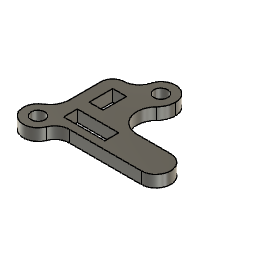
part_A25 (Autodesk Fusion 360 design; units mm, degrees)
Autodesk Fusion 360 part; units mm, degrees
sketch "Sketch1" plane through (0, 0, 0) normal (0, 0, 1) x (1, 0, 0)
  line L0 (0, 0) -> (35, 0)
  line L1 (35, 0) -> (35, 40)
  line L2 (35, 40) -> (0, 40)
  line L3 (0, 40) -> (0, 0)
  dimension "d1" = 35
  dimension "d2" = 40
  constraint horizontal L0
  constraint vertical L1
  constraint horizontal L2
  constraint vertical L3
  constraint coincident L0.start L3.end
  measures "d1" distance of L0.start L0.end
  measures "d2" distance of L0.start L2.end
extrude "Extrude1" add sketch "Sketch1" along normal blind 3
sketch "Sketch2" plane through (0, 0, 3) normal (0, 0, 1) x (-1, 0, 0)
  line L0 (0, -40) -> (0, 0)
  line L1 (0, 0) -> (-35, 0)
  line L2 (-35, 0) -> (-35, -40)
  line L3 (-35, -40) -> (0, -40)
  circle A0 centre (-3.75, -3.75) radius 1.75
  dimension "d5" = 3.5
  dimension "d6" = 3.75
  dimension "d7" = 3.75
  measures "d5" diameter of A0
  measures "d6" distance of L0 A0.centre
  measures "d7" distance of L1 A0.centre
extrude "Extrude2" cut sketch "Sketch2" against normal blind 3 contours A0
fillet "Fillet1" radius 3.75 1 edges at (0, 0, 1.5)
sketch "Sketch3" plane through (0, 0, 3) normal (0, 0, 1) x (-1, 0, 0)
  arc A0 (0, -3.75) -> (-3.75, 0) centre (-3.75, -3.75) ccw
  line L0 (-3.75, 0) -> (-35, 0)
  line L1 (-35, 0) -> (-35, -40)
  line L2 (-35, -40) -> (0, -40)
  line L3 (0, -40) -> (0, -3.75)
  circle A1 centre (-3.75, -3.75) radius 1.75
  line L4 (-7.25, -10.25) -> (-17.75, -10.25)
  line L5 (-17.75, -10.25) -> (-17.75, -6.75)
  line L6 (-17.75, -6.75) -> (-7.25, -6.75)
  line L7 (-7.25, -6.75) -> (-7.25, -10.25)
  dimension "d12" = 10.5
  dimension "d13" = 3.5
  dimension "d14" = 3
  dimension "d15" = 3.5
  constraint horizontal L4
  constraint vertical L5
  constraint horizontal L6
  constraint vertical L7
  measures "d12" distance of L4.start L4.end
  measures "d13" distance of L4.start L6.end
  measures "d14" distance of A0.centre L6
  measures "d15" distance of A0.centre L7
extrude "Extrude3" cut sketch "Sketch3" against normal blind 3 contours L4 L5 L6 L7
sketch "Sketch4" plane through (0, 0, 3) normal (0, 0, 1) x (-1, 0, 0)
  line L0 (-17.75, -10.25) -> (-17.75, -6.75)
  line L1 (-17.75, -6.75) -> (-7.25, -6.75)
  line L2 (-7.25, -6.75) -> (-7.25, -10.25)
  line L3 (-7.25, -10.25) -> (-17.75, -10.25)
  arc A0 (0, -3.75) -> (-3.75, 0) centre (-3.75, -3.75) ccw
  line L4 (-3.75, 0) -> (-35, 0)
  line L5 (-35, 0) -> (-35, -40)
  line L6 (-35, -40) -> (0, -40)
  line L7 (0, -40) -> (0, -3.75)
  circle A1 centre (-3.75, -3.75) radius 1.75
  line L8 (-7.25, -13.25) -> (-10.75, -13.25)
  line L9 (-10.75, -13.25) -> (-10.75, -19.25)
  line L10 (-10.75, -19.25) -> (-7.25, -19.25)
  line L11 (-7.25, -19.25) -> (-7.25, -13.25)
  dimension "d18" = 3.5
  dimension "d19" = 6
  dimension "d20" = 0
  dimension "d21" = 3
  constraint horizontal L8
  constraint vertical L9
  constraint horizontal L10
  constraint vertical L11
  measures "d18" distance of L8.start L8.end
  measures "d19" distance of L8.start L10.end
  measures "d20" distance of L2 L11
  measures "d21" distance of L3 L8
extrude "Extrude4" cut sketch "Sketch4" against normal blind 3 contours L8 L9 L10 L11
sketch "Sketch5" plane through (0, 0, 3) normal (0, 0, 1) x (-1, 0, 0)
  line L0 (-10.75, -13.25) -> (-7.25, -13.25)
  line L1 (-7.25, -13.25) -> (-7.25, -19.25)
  line L2 (-7.25, -19.25) -> (-10.75, -19.25)
  line L3 (-10.75, -19.25) -> (-10.75, -13.25)
  line L4 (-17.75, -10.25) -> (-17.75, -6.75)
  line L5 (-17.75, -6.75) -> (-7.25, -6.75)
  line L6 (-7.25, -6.75) -> (-7.25, -10.25)
  line L7 (-7.25, -10.25) -> (-17.75, -10.25)
  arc A0 (0, -3.75) -> (-3.75, 0) centre (-3.75, -3.75) ccw
  line L8 (-3.75, 0) -> (-35, 0)
  line L9 (-35, 0) -> (-35, -40)
  line L10 (-35, -40) -> (0, -40)
  line L11 (0, -40) -> (0, -3.75)
  circle A1 centre (-3.75, -3.75) radius 1.75
  circle A2 centre (-14.5, -24.25) radius 1.75
  dimension "d24" = 3.5
  dimension "d25" = 5
  dimension "d26" = 3.75
  measures "d24" diameter of A2
  measures "d25" distance of L2 A2.centre
  measures "d26" distance of L3 A2.centre
extrude "Extrude5" cut sketch "Sketch5" against normal blind 3 contours A2
sketch "Sketch8" plane through (0, 0, 3) normal (0, 0, 1) x (-1, 0, 0)
  circle A0 centre (-14.5, -24.25) radius 1.75
  line L0 (-10.75, -13.25) -> (-7.25, -13.25)
  line L1 (-7.25, -13.25) -> (-7.25, -19.25)
  line L2 (-7.25, -19.25) -> (-10.75, -19.25)
  line L3 (-10.75, -19.25) -> (-10.75, -13.25)
  line L4 (-17.75, -10.25) -> (-17.75, -6.75)
  line L5 (-17.75, -6.75) -> (-7.25, -6.75)
  line L6 (-7.25, -6.75) -> (-7.25, -10.25)
  line L7 (-7.25, -10.25) -> (-17.75, -10.25)
  arc A1 (0, -3.75) -> (-3.75, 0) centre (-3.75, -3.75) ccw
  line L8 (-3.75, 0) -> (-35, 0)
  line L9 (-35, 0) -> (-35, -40)
  line L10 (-35, -40) -> (0, -40)
  line L11 (0, -40) -> (0, -3.75)
  circle A2 centre (-3.75, -3.75) radius 1.75
  line L12 (0, -7.5) -> (-4.25, -7.5)
  line L13 (-4.25, -7.5) -> (-4.25, -22.25)
  line L14 (-4.25, -22.25) -> (0, -22.25)
  line L15 (0, -22.25) -> (0, -7.5)
  dimension "d30" = 3.75
  dimension "d31" = 3
  dimension "d32" = 3
  constraint horizontal L12
  constraint vertical L13
  constraint horizontal L14
  constraint vertical L15
  constraint coincident L11 L12.start
  measures "d30" distance of A1.centre L12
  measures "d31" distance of L6 L13
  measures "d32" distance of L2 L14
extrude "Extrude6" cut sketch "Sketch8" against normal blind 3 contours L11 L12 L13 L14 L15
fillet "Fillet2" radius 3.75 1 edges at (0, 7.5, 1.5)
fillet "Fillet3" radius 5 1 edges at (4.25, 7.5, 1.5)
sketch "Sketch9" plane through (0, 0, 3) normal (0, 0, 1) x (-1, 0, 0)
  arc A0 (-1.8214, -6.9661) -> (-3.75, 0) centre (-3.75, -3.75) ccw
  line L0 (-3.75, 0) -> (-35, 0)
  line L1 (-35, 0) -> (-35, -40)
  line L2 (-35, -40) -> (0, -40)
  line L3 (0, -40) -> (0, -22.25)
  line L4 (0, -22.25) -> (-4.25, -22.25)
  line L5 (-4.25, -22.25) -> (-4.25, -11.2542)
  arc A1 (-1.8214, -6.9661) -> (-4.25, -11.2542) centre (0.75, -11.2542) ccw
  circle A2 centre (-3.75, -3.75) radius 1.75
  line L6 (-17.75, -10.25) -> (-17.75, -6.75)
  line L7 (-17.75, -6.75) -> (-7.25, -6.75)
  line L8 (-7.25, -6.75) -> (-7.25, -10.25)
  line L9 (-7.25, -10.25) -> (-17.75, -10.25)
  line L10 (-10.75, -13.25) -> (-7.25, -13.25)
  line L11 (-7.25, -13.25) -> (-7.25, -19.25)
  line L12 (-7.25, -19.25) -> (-10.75, -19.25)
  line L13 (-10.75, -19.25) -> (-10.75, -13.25)
  circle A3 centre (-14.5, -24.25) radius 1.75
  line L14 (0, -22.25) -> (-10.75, -22.25)
  line L15 (-10.75, -22.25) -> (-10.75, -27)
  line L16 (-10.75, -27) -> (0, -27)
  line L17 (0, -27) -> (0, -22.25)
  dimension "d39" = 3.75
  constraint horizontal L14
  constraint vertical L15
  constraint horizontal L16
  constraint vertical L17
  constraint coincident L3.end L4.start
  measures "d39" distance of A3.centre L15
extrude "Extrude7" cut sketch "Sketch9" against normal blind 3 contours L3 L4 L14 L15 L16 L17
fillet "Fillet4" radius 3 1 edges at (4.25, 22.25, 1.5)
sketch "Sketch12" plane through (0, 0, 3) normal (0, 0, 1) x (-1, 0, 0)
  arc A0 (-7.25, -22.25) -> (-4.25, -19.25) centre (-7.25, -19.25) ccw
  line L0 (-4.25, -19.25) -> (-4.25, -11.2542)
  arc A1 (-1.8214, -6.9661) -> (-4.25, -11.2542) centre (0.75, -11.2542) ccw
  arc A2 (-1.8214, -6.9661) -> (-3.75, 0) centre (-3.75, -3.75) ccw
  line L1 (-3.75, 0) -> (-35, 0)
  line L2 (-35, 0) -> (-35, -40)
  line L3 (-35, -40) -> (0, -40)
  line L4 (0, -40) -> (0, -27)
  line L5 (0, -27) -> (-10.75, -27)
  line L6 (-10.75, -27) -> (-10.75, -22.25)
  line L7 (-10.75, -22.25) -> (-7.25, -22.25)
  circle A3 centre (-14.5, -24.25) radius 1.75
  line L8 (-10.75, -13.25) -> (-7.25, -13.25)
  line L9 (-7.25, -13.25) -> (-7.25, -19.25)
  line L10 (-7.25, -19.25) -> (-10.75, -19.25)
  line L11 (-10.75, -19.25) -> (-10.75, -13.25)
  line L12 (-17.75, -10.25) -> (-17.75, -6.75)
  line L13 (-17.75, -6.75) -> (-7.25, -6.75)
  line L14 (-7.25, -6.75) -> (-7.25, -10.25)
  line L15 (-7.25, -10.25) -> (-17.75, -10.25)
  circle A4 centre (-3.75, -3.75) radius 1.75
  line L16 (-10.75, -27) -> (0, -27)
  line L17 (0, -27) -> (0, -40)
  line L18 (0, -40) -> (-10.75, -40)
  line L19 (-10.75, -40) -> (-10.75, -27)
  constraint horizontal L16
  constraint vertical L17
  constraint horizontal L18
  constraint vertical L19
  constraint coincident L3.end L4.start
  constraint coincident L5.end L6.start
extrude "Extrude9" cut sketch "Sketch12" against normal blind 3 contours L3 L4 L5 L16 L17 L18 L19
sketch "Sketch13" plane through (0, 0, 3) normal (0, 0, 1) x (-1, 0, 0)
  circle A0 centre (-3.75, -3.75) radius 1.75
  line L0 (-17.75, -10.25) -> (-17.75, -6.75)
  line L1 (-17.75, -6.75) -> (-7.25, -6.75)
  line L2 (-7.25, -6.75) -> (-7.25, -10.25)
  line L3 (-7.25, -10.25) -> (-17.75, -10.25)
  line L4 (-10.75, -13.25) -> (-7.25, -13.25)
  line L5 (-7.25, -13.25) -> (-7.25, -19.25)
  line L6 (-7.25, -19.25) -> (-10.75, -19.25)
  line L7 (-10.75, -19.25) -> (-10.75, -13.25)
  circle A1 centre (-14.5, -24.25) radius 1.75
  line L8 (-10.75, -40) -> (-10.75, -22.25)
  line L9 (-10.75, -22.25) -> (-7.25, -22.25)
  arc A2 (-7.25, -22.25) -> (-4.25, -19.25) centre (-7.25, -19.25) ccw
  line L10 (-4.25, -19.25) -> (-4.25, -11.2542)
  arc A3 (-1.8214, -6.9661) -> (-4.25, -11.2542) centre (0.75, -11.2542) ccw
  arc A4 (-1.8214, -6.9661) -> (-3.75, 0) centre (-3.75, -3.75) ccw
  line L11 (-3.75, 0) -> (-35, 0)
  line L12 (-35, 0) -> (-35, -40)
  line L13 (-35, -40) -> (-10.75, -40)
  line L14 (-35, -40) -> (-18.25, -40)
  line L15 (-18.25, -40) -> (-18.25, -22.25)
  line L16 (-18.25, -22.25) -> (-35, -22.25)
  line L17 (-35, -22.25) -> (-35, -40)
  dimension "d48" = 3.75
  constraint horizontal L14
  constraint vertical L15
  constraint horizontal L16
  constraint vertical L17
  constraint coincident L12.end L13.start
  measures "d48" distance of A1.centre L15
extrude "Extrude10" cut sketch "Sketch13" against normal blind 3 contours L12 L13 L14 L15 L16 L17
sketch "Sketch14" plane through (0, 0, 3) normal (0, 0, 1) x (-1, 0, 0)
  line L0 (-35, -22.25) -> (-18.25, -22.25)
  line L1 (-18.25, -22.25) -> (-18.25, -40)
  line L2 (-18.25, -40) -> (-10.75, -40)
  line L3 (-10.75, -40) -> (-10.75, -22.25)
  line L4 (-10.75, -22.25) -> (-7.25, -22.25)
  arc A0 (-7.25, -22.25) -> (-4.25, -19.25) centre (-7.25, -19.25) ccw
  line L5 (-4.25, -19.25) -> (-4.25, -11.2542)
  arc A1 (-1.8214, -6.9661) -> (-4.25, -11.2542) centre (0.75, -11.2542) ccw
  arc A2 (-1.8214, -6.9661) -> (-3.75, 0) centre (-3.75, -3.75) ccw
  line L6 (-3.75, 0) -> (-35, 0)
  line L7 (-35, 0) -> (-35, -22.25)
  circle A3 centre (-14.5, -24.25) radius 1.75
  line L8 (-10.75, -13.25) -> (-7.25, -13.25)
  line L9 (-7.25, -13.25) -> (-7.25, -19.25)
  line L10 (-7.25, -19.25) -> (-10.75, -19.25)
  line L11 (-10.75, -19.25) -> (-10.75, -13.25)
  line L12 (-17.75, -10.25) -> (-17.75, -6.75)
  line L13 (-17.75, -6.75) -> (-7.25, -6.75)
  line L14 (-7.25, -6.75) -> (-7.25, -10.25)
  line L15 (-7.25, -10.25) -> (-17.75, -10.25)
  circle A4 centre (-3.75, -3.75) radius 1.75
  line L16 (-10.75, -40) -> (-18.25, -40)
  line L17 (-18.25, -40) -> (-18.25, -28)
  line L18 (-18.25, -28) -> (-10.75, -28)
  line L19 (-10.75, -28) -> (-10.75, -40)
  dimension "d51" = 3.75
  constraint horizontal L16
  constraint vertical L17
  constraint horizontal L18
  constraint vertical L19
  constraint coincident L1 L17.end
  constraint coincident L2.end L3.start
  measures "d51" distance of A3.centre L18
extrude "Extrude11" cut sketch "Sketch14" against normal blind 3 contours L1 L2 L3 L16 L17 L18 L19
fillet "Fillet5" radius 3.75 1 edges at (10.75, 28, 1.5)
fillet "Fillet6" radius 3.75 1 edges at (18.25, 28, 1.5)
sketch "Sketch15" plane through (0, 0, 3) normal (0, 0, 1) x (-1, 0, 0)
  circle A0 centre (-3.75, -3.75) radius 1.75
  line L0 (-17.75, -10.25) -> (-17.75, -6.75)
  line L1 (-17.75, -6.75) -> (-7.25, -6.75)
  line L2 (-7.25, -6.75) -> (-7.25, -10.25)
  line L3 (-7.25, -10.25) -> (-17.75, -10.25)
  line L4 (-10.75, -13.25) -> (-7.25, -13.25)
  line L5 (-7.25, -13.25) -> (-7.25, -19.25)
  line L6 (-7.25, -19.25) -> (-10.75, -19.25)
  line L7 (-10.75, -19.25) -> (-10.75, -13.25)
  circle A1 centre (-14.5, -24.25) radius 1.75
  arc A2 (-18.25, -24.25) -> (-10.75, -24.25) centre (-14.5, -24.25) ccw
  line L8 (-10.75, -24.25) -> (-10.75, -22.25)
  line L9 (-10.75, -22.25) -> (-7.25, -22.25)
  arc A3 (-7.25, -22.25) -> (-4.25, -19.25) centre (-7.25, -19.25) ccw
  line L10 (-4.25, -19.25) -> (-4.25, -11.2542)
  arc A4 (-1.8214, -6.9661) -> (-4.25, -11.2542) centre (0.75, -11.2542) ccw
  arc A5 (-1.8214, -6.9661) -> (-3.75, 0) centre (-3.75, -3.75) ccw
  line L11 (-3.75, 0) -> (-35, 0)
  line L12 (-35, 0) -> (-35, -22.25)
  line L13 (-35, -22.25) -> (-18.25, -22.25)
  line L14 (-18.25, -22.25) -> (-18.25, -24.25)
  line L15 (-7.5, 0) -> (-35, 0)
  line L16 (-35, 0) -> (-35, -4.75)
  line L17 (-35, -4.75) -> (-7.5, -4.75)
  line L18 (-7.5, -4.75) -> (-7.5, 0)
  dimension "d58" = 2
  dimension "d59" = 3.75
  constraint horizontal L15
  constraint vertical L16
  constraint horizontal L17
  constraint vertical L18
  constraint coincident L12 L16.end
  constraint coincident L11 L15.start
  measures "d58" distance of L1 L17
  measures "d59" distance of A0.centre L18
extrude "Extrude12" cut sketch "Sketch15" against normal blind 3 contours L11 L12 L15 L16 L17 L18
fillet "Fillet7" radius 3.75 1 edges at (7.5, 0, 1.5)
fillet "Fillet8" radius 3.75 1 edges at (7.5, 4.75, 1.5)
sketch "Sketch16" plane through (0, 0, 3) normal (0, 0, 1) x (-1, 0, 0)
  circle A0 centre (-14.5, -24.25) radius 1.75
  line L0 (-10.75, -13.25) -> (-7.25, -13.25)
  line L1 (-7.25, -13.25) -> (-7.25, -19.25)
  line L2 (-7.25, -19.25) -> (-10.75, -19.25)
  line L3 (-10.75, -19.25) -> (-10.75, -13.25)
  line L4 (-17.75, -10.25) -> (-17.75, -6.75)
  line L5 (-17.75, -6.75) -> (-7.25, -6.75)
  line L6 (-7.25, -6.75) -> (-7.25, -10.25)
  line L7 (-7.25, -10.25) -> (-17.75, -10.25)
  circle A1 centre (-3.75, -3.75) radius 1.75
  arc A2 (-10.7276, -4.75) -> (-7.2388, -2.375) centre (-10.7276, -1) ccw
  line L8 (-10.7276, -4.75) -> (-35, -4.75)
  line L9 (-35, -4.75) -> (-35, -22.25)
  line L10 (-35, -22.25) -> (-18.25, -22.25)
  line L11 (-18.25, -22.25) -> (-18.25, -24.25)
  arc A3 (-18.25, -24.25) -> (-10.75, -24.25) centre (-14.5, -24.25) ccw
  line L12 (-10.75, -24.25) -> (-10.75, -22.25)
  line L13 (-10.75, -22.25) -> (-7.25, -22.25)
  arc A4 (-7.25, -22.25) -> (-4.25, -19.25) centre (-7.25, -19.25) ccw
  line L14 (-4.25, -19.25) -> (-4.25, -11.2542)
  arc A5 (-1.8214, -6.9661) -> (-4.25, -11.2542) centre (0.75, -11.2542) ccw
  arc A6 (-1.8214, -6.9661) -> (-7.2388, -2.375) centre (-3.75, -3.75) ccw
  line L15 (-32.75, -4.75) -> (-35, -4.75)
  line L16 (-35, -4.75) -> (-35, -22.25)
  line L17 (-35, -22.25) -> (-32.75, -22.25)
  line L18 (-32.75, -22.25) -> (-32.75, -4.75)
  dimension "d66" = 15
  constraint horizontal L15
  constraint vertical L16
  constraint horizontal L17
  constraint vertical L18
  constraint coincident L9.end L10.start
  constraint coincident L8 L15.start
  measures "d66" distance of L4 L18
extrude "Extrude13" cut sketch "Sketch16" against normal blind 3 contours L8 L9 L10 L15 L16 L17 L18
sketch "Sketch17" plane through (0, 0, 3) normal (0, 0, 1) x (-1, 0, 0)
  line L0 (-32.75, -4.75) -> (-32.75, -22.25)
  line L1 (-32.75, -22.25) -> (-18.25, -22.25)
  line L2 (-18.25, -22.25) -> (-18.25, -24.25)
  arc A0 (-18.25, -24.25) -> (-10.75, -24.25) centre (-14.5, -24.25) ccw
  line L3 (-10.75, -24.25) -> (-10.75, -22.25)
  line L4 (-10.75, -22.25) -> (-7.25, -22.25)
  arc A1 (-7.25, -22.25) -> (-4.25, -19.25) centre (-7.25, -19.25) ccw
  line L5 (-4.25, -19.25) -> (-4.25, -11.2542)
  arc A2 (-1.8214, -6.9661) -> (-4.25, -11.2542) centre (0.75, -11.2542) ccw
  arc A3 (-1.8214, -6.9661) -> (-7.2388, -2.375) centre (-3.75, -3.75) ccw
  arc A4 (-10.7276, -4.75) -> (-7.2388, -2.375) centre (-10.7276, -1) ccw
  line L6 (-10.7276, -4.75) -> (-32.75, -4.75)
  circle A5 centre (-14.5, -24.25) radius 1.75
  line L7 (-10.75, -13.25) -> (-7.25, -13.25)
  line L8 (-7.25, -13.25) -> (-7.25, -19.25)
  line L9 (-7.25, -19.25) -> (-10.75, -19.25)
  line L10 (-10.75, -19.25) -> (-10.75, -13.25)
  line L11 (-17.75, -10.25) -> (-17.75, -6.75)
  line L12 (-17.75, -6.75) -> (-7.25, -6.75)
  line L13 (-7.25, -6.75) -> (-7.25, -10.25)
  line L14 (-7.25, -10.25) -> (-17.75, -10.25)
  circle A6 centre (-3.75, -3.75) radius 1.75
  line L15 (-32.75, -22.25) -> (-18.25, -22.25)
  line L16 (-18.25, -22.25) -> (-18.25, -12.25)
  line L17 (-18.25, -12.25) -> (-32.75, -12.25)
  line L18 (-32.75, -12.25) -> (-32.75, -22.25)
  dimension "d69" = 2
  constraint horizontal L15
  constraint vertical L16
  constraint horizontal L17
  constraint vertical L18
  constraint coincident L0.end L1.start
  measures "d69" distance of L14 L17
extrude "Extrude14" cut sketch "Sketch17" against normal blind 3 contours L0 L1 L15 L16 L17 L18
fillet "Fillet9" radius 3.75 1 edges at (32.75, 12.25, 1.5)
fillet "Fillet10" radius 3.75 1 edges at (32.75, 4.75, 1.5)
sketch "Sketch18" plane through (0, 0, 3) normal (0, 0, 1) x (-1, 0, 0)
  arc A0 (-29, -4.75) -> (-29, -12.25) centre (-29, -8.5) ccw
  line L0 (-29, -12.25) -> (-18.25, -12.25)
  line L1 (-18.25, -12.25) -> (-18.25, -24.25)
  arc A1 (-18.25, -24.25) -> (-10.75, -24.25) centre (-14.5, -24.25) ccw
  line L2 (-10.75, -24.25) -> (-10.75, -22.25)
  line L3 (-10.75, -22.25) -> (-7.25, -22.25)
  arc A2 (-7.25, -22.25) -> (-4.25, -19.25) centre (-7.25, -19.25) ccw
  line L4 (-4.25, -19.25) -> (-4.25, -11.2542)
  arc A3 (-1.8214, -6.9661) -> (-4.25, -11.2542) centre (0.75, -11.2542) ccw
  arc A4 (-1.8214, -6.9661) -> (-7.2388, -2.375) centre (-3.75, -3.75) ccw
  arc A5 (-10.7276, -4.75) -> (-7.2388, -2.375) centre (-10.7276, -1) ccw
  line L5 (-10.7276, -4.75) -> (-29, -4.75)
  circle A6 centre (-14.5, -24.25) radius 1.75
  line L6 (-10.75, -13.25) -> (-7.25, -13.25)
  line L7 (-7.25, -13.25) -> (-7.25, -19.25)
  line L8 (-7.25, -19.25) -> (-10.75, -19.25)
  line L9 (-10.75, -19.25) -> (-10.75, -13.25)
  line L10 (-17.75, -10.25) -> (-17.75, -6.75)
  line L11 (-17.75, -6.75) -> (-7.25, -6.75)
  line L12 (-7.25, -6.75) -> (-7.25, -10.25)
  line L13 (-7.25, -10.25) -> (-17.75, -10.25)
  circle A7 centre (-3.75, -3.75) radius 1.75
  line L14 (-18.25, -12.25) -> (-12.75, -12.25)
  line L15 (-12.75, -12.25) -> (-12.75, -19.25)
  line L16 (-12.75, -19.25) -> (-18.25, -19.25)
  line L17 (-18.25, -19.25) -> (-18.25, -12.25)
  dimension "d76" = 2
  constraint horizontal L14
  constraint vertical L15
  constraint horizontal L16
  constraint vertical L17
  constraint coincident L0.end L1.start
  measures "d76" distance of L9 L15
extrude "Extrude15" cut sketch "Sketch18" against normal blind 3 contours L1 L14 L15 L16 L17
fillet "Fillet11" radius 5 1 edges at (18.25, 19.25, 1.5)
fillet "Fillet12" radius 5 1 edges at (12.75, 19.25, 1.5)
fillet "Fillet13" radius 5 1 edges at (12.75, 12.25, 1.5)
fillet "Fillet14" radius 4 1 edges at (10.75, 22.25, 1.5)
